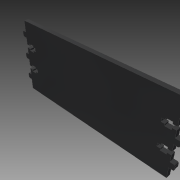
# Autodesk Inventor part: front_panel_2004_bottom
Saved by Autodesk Inventor 2014 (Build 180170000, 170)
## iProperties
Created: 2014-01-11
Part Number: front_panel_2004_bottom
Material: Generic
Document SubType Name: Modeling
Designer: buben
Density: 1 g/cm^3
Appearance: Anodized - Dark Gray
Author: buben
Autodesk Inventor part; units mm, degrees
ref_plane "YZ Plane" through (0, 0, 0) normal (1, 0, 0) x (0, 1, 0)
ref_plane "XZ Plane" through (0, 0, 0) normal (0, 1, 0) x (-1, 0, 0)
ref_plane "XY Plane" through (0, 0, 0) normal (0, 0, 1) x (1, 0, 0)
sketch "Sketch1" plane through (0, 0, 0) normal (0, 1, 0) x (-1, 0, 0)
  line L0 (0, 0) -> (220, 0)
  line L1 (220, 0) -> (220, 100)
  line L2 (220, 100) -> (0, 100)
  line L3 (0, 100) -> (0, 0)
  dimension "d11" = 220
  dimension "d16" = 100
  constraints: 8 end point, 2 parallel, 1 horizontal, 1 perpendicular
  measures "d11" distance of L0.start L0.end
  measures "d16" distance of L2.end L0.start
extrude "Extrusion3" add sketch "Sketch1" along normal blind 6
sketch "Sketch3" plane through (0, 0, 0) normal (0, -1, 0) x (1, 0, 0)
  line L0 (0, 100) -> (0, 0) projected
  line L1 (-220, 0) -> (-220, 100) projected
  line L2 (-220, 85) -> (-224, 85)
  line L3 (-226, 83) -> (-226, 79)
  line L4 (-224, 77) -> (-220, 77)
  line L5 (-220, 77) -> (-220, 85)
  line L6 (-220, 54) -> (-224, 54)
  line L7 (-226, 52) -> (-226, 48)
  line L8 (-224, 46) -> (-220, 46)
  line L9 (-220, 46) -> (-220, 54)
  line L10 (-220, 23) -> (-224, 23)
  line L11 (-226, 21) -> (-226, 17)
  line L12 (-224, 15) -> (-220, 15)
  line L13 (-220, 15) -> (-220, 23)
  line L14 (0, 85) -> (4, 85)
  line L15 (6, 83) -> (6, 79)
  line L16 (4, 77) -> (0, 77)
  line L17 (0, 77) -> (0, 85)
  line L18 (0, 54) -> (4, 54)
  line L19 (6, 52) -> (6, 48)
  line L20 (4, 46) -> (0, 46)
  line L21 (0, 46) -> (0, 54)
  line L22 (0, 23) -> (4, 23)
  line L23 (6, 21) -> (6, 17)
  line L24 (4, 15) -> (0, 15)
  line L25 (0, 15) -> (0, 23)
  arc A0 (-224, 85) -> (-226, 83) centre (-224, 83) ccw
  arc A1 (-226, 79) -> (-224, 77) centre (-224, 79) ccw
  arc A2 (-224, 54) -> (-226, 52) centre (-224, 52) ccw
  arc A3 (-226, 48) -> (-224, 46) centre (-224, 48) ccw
  arc A4 (-224, 23) -> (-226, 21) centre (-224, 21) ccw
  arc A5 (-226, 17) -> (-224, 15) centre (-224, 17) ccw
  arc A6 (6, 83) -> (4, 85) centre (4, 83) ccw
  arc A7 (4, 77) -> (6, 79) centre (4, 79) ccw
  arc A8 (6, 52) -> (4, 54) centre (4, 52) ccw
  arc A9 (4, 46) -> (6, 48) centre (4, 48) ccw
  arc A10 (6, 21) -> (4, 23) centre (4, 21) ccw
  arc A11 (4, 15) -> (6, 17) centre (4, 17) ccw
  line L26 (-222, 77) -> (-222, 54) construction
  line L27 (-222, 23) -> (-222, 46) construction
  point P0 (-226, 50)
  point P1 (-220, 50)
  dimension "d35" = 2
  dimension "d36" = 8
  dimension "d37" = 6
  dimension "d38" = 8
  dimension "d39" = 8
  dimension "d40" = 8
  dimension "d41" = 8
  dimension "d42" = 8
  dimension "d43" = 6
  dimension "d44" = 23
  constraints: 52 end point, 24 point on circle, 24 tangent, 12 centre point, 12 parallel, 11 equal radius, 8 collinear, 6 horizontal, 6 midpoint, 6 perpendicular, 6 point on line, 1 horizontal alignment
  measures "d35" radius of A0
  measures "d36" distance between parallel lines of L4 L2
  measures "d37" distance between parallel lines of L5 L3
  measures "d38" distance between parallel lines of L8 L6
  measures "d39" distance between parallel lines of L12 L10
  measures "d40" distance between parallel lines of L16 L14
  measures "d41" distance between parallel lines of L20 L18
  measures "d42" distance between parallel lines of L24 L22
  measures "d43" distance from line of L0 L15.end
  measures "d44" distance of L26.start L26.end
extrude "Extrusion4" add sketch "Sketch3" against normal blind 6
sketch "Sketch4" plane through (0, 0, 0) normal (0, -1, 0) x (1, 0, 0)
  line L0 (0, 0) -> (-220, 0) projected
  line L1 (-220, 100) -> (0, 100) projected
  line L2 (-220, 54) -> (-220, 77) projected
  line L3 (-220, 23) -> (-220, 46) projected
  line L4 (-203.7, 67.75) -> (-203.7, 63.25)
  line L5 (-220, 63.25) -> (-220, 67.75)
  line L6 (-215, 70.25) -> (-207.7, 70.25)
  line L7 (-207.7, 60.75) -> (-215, 60.75)
  line L8 (-220, 67.75) -> (-215, 67.75)
  line L9 (-207.7, 67.75) -> (-203.7, 67.75)
  line L10 (-203.7, 63.25) -> (-207.7, 63.25)
  line L11 (-215, 63.25) -> (-220, 63.25)
  line L12 (-215, 60.75) -> (-215, 63.25)
  line L13 (-215, 67.75) -> (-215, 70.25)
  line L14 (-207.7, 70.25) -> (-207.7, 67.75)
  line L15 (-207.7, 63.25) -> (-207.7, 60.75)
  line L16 (-203.7, 36.75) -> (-203.7, 32.25)
  line L17 (-220, 32.25) -> (-220, 36.75)
  line L18 (-215, 39.25) -> (-207.7, 39.25)
  line L19 (-207.7, 29.75) -> (-215, 29.75)
  line L20 (-220, 36.75) -> (-215, 36.75)
  line L21 (-207.7, 36.75) -> (-203.7, 36.75)
  line L22 (-203.7, 32.25) -> (-207.7, 32.25)
  line L23 (-215, 32.25) -> (-220, 32.25)
  line L24 (-215, 29.75) -> (-215, 32.25)
  line L25 (-215, 36.75) -> (-215, 39.25)
  line L26 (-207.7, 39.25) -> (-207.7, 36.75)
  line L27 (-207.7, 32.25) -> (-207.7, 29.75)
  line L28 (-110, 100) -> (-110, 0) construction
  line L29 (-16.3, 67.75) -> (-16.3, 63.25)
  line L30 (0, 63.25) -> (0, 67.75)
  line L31 (-5, 70.25) -> (-12.3, 70.25)
  line L32 (-12.3, 60.75) -> (-5, 60.75)
  line L33 (0, 67.75) -> (-5, 67.75)
  line L34 (-12.3, 67.75) -> (-16.3, 67.75)
  line L35 (-16.3, 63.25) -> (-12.3, 63.25)
  line L36 (-5, 63.25) -> (0, 63.25)
  line L37 (-5, 60.75) -> (-5, 63.25)
  line L38 (-5, 67.75) -> (-5, 70.25)
  line L39 (-12.3, 70.25) -> (-12.3, 67.75)
  line L40 (-12.3, 63.25) -> (-12.3, 60.75)
  line L41 (0, 36.75) -> (-5, 36.75)
  line L42 (-16.3, 36.75) -> (-16.3, 32.25)
  line L43 (-16.3, 32.25) -> (-12.3, 32.25)
  line L44 (-12.3, 32.25) -> (-12.3, 29.75)
  line L45 (-12.3, 39.25) -> (-12.3, 36.75)
  line L46 (-12.3, 29.75) -> (-5, 29.75)
  line L47 (-5, 29.75) -> (-5, 32.25)
  line L48 (-5, 36.75) -> (-5, 39.25)
  line L49 (-5, 39.25) -> (-12.3, 39.25)
  line L50 (-5, 32.25) -> (0, 32.25)
  line L51 (0, 32.25) -> (0, 36.75)
  line L52 (-12.3, 36.75) -> (-16.3, 36.75)
  point P0 (-220, 65.5)
  point P1 (-220, 34.5)
  point P2 (0, 65.5)
  point P3 (0, 34.5)
  dimension "d47" = 4.5
  dimension "d48" = 2.5
  dimension "d49" = 2.5
  dimension "d50" = 5
  dimension "d51" = 4
  dimension "d52" = 7.3
  dimension "d53" = 4.5
  dimension "d54" = 2.5
  dimension "d55" = 2.5
  dimension "d56" = 5
  dimension "d57" = 4
  dimension "d58" = 7.3
  constraints: 98 end point, 26 symmetric about line, 20 parallel, 8 collinear, 8 perpendicular, 6 horizontal, 6 midpoint
  measures "d47" distance of L4.start L4.end
  measures "d48" distance of L6.end L9.start
  measures "d49" distance of L10.end L7.start
  measures "d50" distance of L5.end L8.end
  measures "d51" distance of L9.start L4.start
  measures "d52" distance of L6.start L6.end
  measures "d53" distance of L16.start L16.end
  measures "d54" distance of L26.start L26.end
  measures "d55" distance of L22.end L27.end
  measures "d56" distance of L20.start L20.end
  measures "d57" distance of L26.end L16.start
  measures "d58" distance of L25.end L26.start
extrude "Extrusion5" cut sketch "Sketch4" against normal through all
equation "\"d38\" = d36"
equation "\"d39\" = d38"
equation "\"d40\" = d36"
equation "\"d41\" = d40"
equation "\"d42\" = d41"
equation "\"d43\" = d37"
equation "\"d49\" = d48"
equation "\"d55\" = d54"
body "Solid2"
